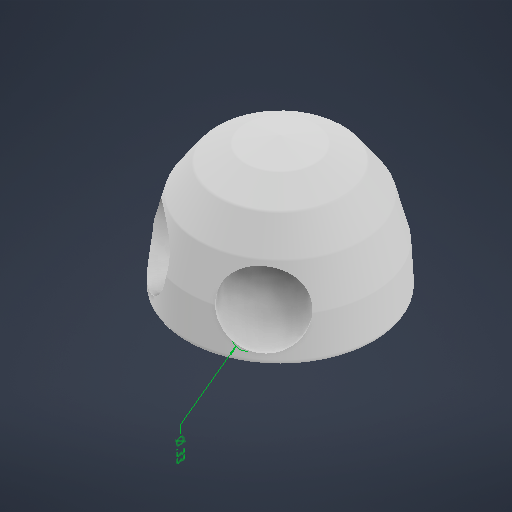
# Autodesk Inventor part: Head
Saved by Autodesk Inventor 2025.2 (Build 292293000, 293)
## iProperties
Created: 2025-03-31
Part Number: Head
Material: Generic
Document SubType Name: Modeling
Designer: mylap
Density: 1 g/cm^3
Appearance: Default
Author: mylap
## iProperties of the stored document Head_3DPrint.ipt
Created: 2025-03-31
Part Number: Head_3DPrint
Material: Generic
Document SubType Name: Modeling
Designer: mylap
Density: 1 g/cm^3
Appearance: Default
Author: mylap
Autodesk Inventor part; units mm, degrees
ref_plane "XZ Plane" through (0, 0, 0) normal (0, 1, 0) x (-1, 0, 0)
sketch "Sketch1" plane through (0, 0, 0) normal (0, 0, 1) x (1, 0, 0)
  line L0 (1.9155, 84.5388) -> (46.3655, 84.5388) construction
  line L1 (46.3655, 84.5388) -> (46.3655, 1.9888) construction
  line L2 (46.3655, 1.9888) -> (1.9155, 1.9888) construction
  line L3 (1.9155, 1.9888) -> (1.9155, 84.5388) construction
  line L4 (13.0242, 66.1379) -> (35.273, 66.1379)
  line L5 (13.0242, 66.1379) -> (13.304, 71.2552)
  line L6 (13.304, 71.2552) -> (14.5683, 76.0081)
  line L7 (14.5683, 76.0081) -> (16.9096, 79.3562)
  line L8 (16.9096, 79.3562) -> (20.1875, 81.1824)
  line L9 (20.1875, 81.1824) -> (24.3082, 82.0721)
  line L10 (24.3082, 82.0721) -> (24.3082, 66.1379)
  line L11 (35.5922, 66.1379) -> (35.3124, 71.2552)
  line L12 (35.3124, 71.2552) -> (34.0481, 76.0081)
  line L13 (34.0481, 76.0081) -> (31.7068, 79.3562)
  line L14 (31.7068, 79.3562) -> (28.4289, 81.1824)
  line L15 (28.4289, 81.1824) -> (24.3082, 82.0721)
  point P0 (0, 0)
  constraints: 24 end point, 5 symmetric about line, 1 horizontal, 1 perpendicular, 1 point on line, 2 other
revolve "Revolution1" add sketch "Sketch1" angle 360 about axis through (24.3082, 82.0721, 0) along (0, -1, 0)
fillet "Fillet1" radius 0.635 5 edges at (35.5922, 66.1379, 0) (35.3124, 71.2552, 0) (34.0481, 76.0081, 0) (31.7068, 79.3562, 0) (28.4289, 81.1824, 0)
ref_plane "Work Plane1" through (0, 0, 7.9375) normal (0, 0, 1) x (1, 0, 0)
sketch "Sketch2" plane through (0, 0, 7.9375) normal (0, 0, 1) x (1, 0, 0)
  line L0 (1.9442, 84.5823) -> (46.3942, 84.5823) construction
  line L1 (46.3942, 84.5823) -> (46.3942, 2.0323) construction
  line L2 (46.3942, 2.0323) -> (1.9442, 2.0323) construction
  line L3 (1.9442, 2.0323) -> (1.9442, 84.5823) construction
  circle A0 centre (18.1243, 71.3329) radius 4.1255
  circle A1 centre (30.3101, 71.3329) radius 4.1275
  line L4 (18.1243, 71.3329) -> (30.3101, 71.3329)
  line L5 (30.3101, 71.3329) -> (34.4376, 71.3329)
  line L6 (18.1243, 71.3329) -> (13.9988, 71.3329)
  point P0 (0, 0)
  point P1 (26.1826, 71.3329)
  point P2 (22.2498, 71.3329)
  dimension "d11" = 8.251
  dimension "d12" = 8.255
  constraints: 6 end point, 2 point on line, 1 horizontal, 8 other
revolve "Revolution2" cut sketch "Sketch2" angle 360 about axis through (18.1243, 71.3329, 7.9375) along (1, 0, 0) picked at (15.4139, 71.662) picked at (28.062, 72.8846) contours L4 L6 A0 | A1 L5 L4
ref_plane "Work Plane2" through (24.3078, 0, 0) normal (1, 0, 0) x (0, 1, 0)
sketch "Sketch3" plane through (24.3078, 0, 0) normal (1, 0, 0) x (0, 1, 0)
  line L0 (83.2138, 13.5179) -> (83.2138, -13.8458) construction
  line L1 (83.2138, -13.8458) -> (60.6921, -13.8458) construction
  line L2 (60.6921, -13.8458) -> (60.6921, 13.5179) construction
  line L3 (60.6921, 13.5179) -> (83.2138, 13.5179) construction
  circle A0 centre (66.0006, -11.3657) radius 0.762
  circle A1 centre (66.0006, -11.3657) radius 0.381
  line L4 (66.1379, -10.6133) -> (66.1379, 10.6133) projected
  line L5 (66.6605, -11.7467) -> (67.213, -11.2252)
  line L6 (71.1899, -11.0078) -> (66.8076, -11.2474) projected
  line L7 (66.1379, -10.0536) -> (66.1379, -10.6133)
  line L8 (67.213, -11.2252) -> (66.7496, -11.2252)
  line L9 (65.5576, -10.7458) -> (66.1379, -10.0864)
  line L10 (66.1379, -10.0864) -> (66.1379, -10.6162)
  arc A2 (67.213, -11.2252) -> (66.1379, -10.0864) centre (66.6755, -10.6558) ccw
  point P0 (0, 0)
  dimension "d19" = 1.524
  dimension "d20" = 0.762
  constraints: 10 end point, 6 point on circle, 4 point on line, 3 centre point, 1 coincident, 1 collinear, 1 perpendicular, 1 tangent, 2 other
  measures "d19" diameter of A0
  measures "d20" diameter of A1
extrude "Extrusion1" add sketch "Sketch3" along normal mid plane 1.143
body "Solid1"
